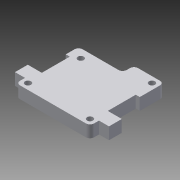
# Autodesk Inventor part: XcrRightTop
Saved by Autodesk Inventor 2013 (Build 170138000, 138)
## iProperties
Created: 2015-01-14
Part Number: XcrRightTop
Material: Generic
Document SubType Name: Modeling
Designer: dzban
Density: 1 g/cm^3
Author: dzban
Autodesk Inventor part; units mm, degrees
ref_plane "YZ Plane" through (0, 0, 0) normal (1, 0, 0) x (0, 1, 0)
ref_plane "XZ Plane" through (0, 0, 0) normal (0, 1, 0) x (-1, 0, 0)
ref_plane "XY Plane" through (0, 0, 0) normal (0, 0, 1) x (1, 0, 0)
sketch "Sketch1" plane through (0, 0, 0) normal (0, 0, 1) x (1, 0, 0)
  arc A0 (-2, 0) -> (0, 2) centre (-2, 2) ccw
  line L0 (0, 4.5) -> (0, 2)
  line L1 (5, 4.5) -> (0, 4.5)
  line L2 (5, 10.9) -> (5, 4.5)
  line L3 (-2, 10.9) -> (5, 10.9)
  line L4 (-2, 24.9) -> (-2, 10.9)
  line L5 (0, 24.9) -> (-2, 24.9)
  line L6 (0, 35) -> (0, 24.9)
  arc A1 (0, 35) -> (-2, 37) centre (-2, 35) ccw
  line L7 (-13, 37) -> (-2, 37)
  arc A2 (-13, 37) -> (-15, 35) centre (-13, 35) ccw
  line L8 (-15, 33.3) -> (-15, 35)
  arc A3 (-17, 31.3) -> (-15, 33.3) centre (-17, 33.3) ccw
  line L9 (-35, 31.3) -> (-17, 31.3)
  arc A4 (-35, 31.3) -> (-37, 29.3) centre (-35, 29.3) ccw
  line L10 (-37, 24.9) -> (-37, 29.3)
  line L11 (-35, 24.9) -> (-37, 24.9)
  line L12 (-35, 10.9) -> (-35, 24.9)
  line L13 (-42, 10.9) -> (-35, 10.9)
  line L14 (-42, 4.5) -> (-42, 10.9)
  line L15 (-37, 4.5) -> (-42, 4.5)
  line L16 (-37, 2) -> (-37, 4.5)
  arc A5 (-37, 2) -> (-35, 0) centre (-35, 2) ccw
  line L17 (-2, 0) -> (-35, 0)
  circle A6 centre (-3, 34) radius 1.5
  circle A7 centre (-34, 3) radius 1.5
  circle A8 centre (-3, 3) radius 1.5
  circle A9 centre (-31.5, 26.9) radius 1.5
  point P0 (0, 0)
  point P1 (0, 0)
  constraints: 36 end point, 12 point on circle, 10 centre point
extrude "Extrusion1" add sketch "Sketch1" along normal blind 6
body "Solid1"
